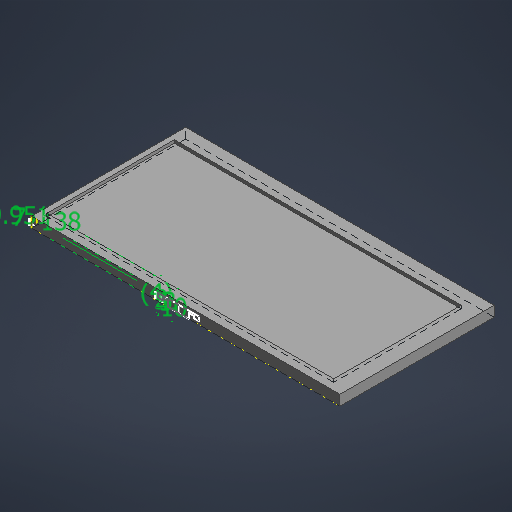
# Autodesk Inventor part: tray_multipart
Saved by Autodesk Inventor 2026 (Build 300175050, 175E)
## iProperties
Part Number: tray_multipart
Material: Generic
Document SubType Name: Modeling
Designer: romanov
Appearance: Default
Author: romanov
Autodesk Inventor part; units mm, degrees
ref_plane "YZ Plane" through (0, 0, 0) normal (1, 0, 0) x (0, 1, 0)
ref_plane "XZ Plane" through (0, 0, 0) normal (0, 1, 0) x (-1, 0, 0)
ref_plane "XY Plane" through (0, 0, 0) normal (0, 0, 1) x (1, 0, 0)
sketch "Sketch1" plane through (0, 0, 0) normal (0, 1, 0) x (-1, 0, 0)
  line L0 (150, 75) -> (-150, 75)
  line L1 (-150, 75) -> (-150, -75)
  line L2 (-150, -75) -> (150, -75)
  line L3 (150, -75) -> (150, 75)
  line L4 (150, 75) -> (-150, -75) construction
  line L5 (-150, 75) -> (150, -75) construction
  point P0 (0, 0)
  dimension "d0" = 300
  dimension "d1" = 150
  constraints: 12 end point, 2 midpoint, 2 parallel, 1 horizontal, 1 perpendicular
  measures "d0" distance between parallel lines of L1 L3
  measures "d1" distance between parallel lines of L0 L2
extrude "Extrusion1" add sketch "Sketch1" along normal blind 10
sketch "Sketch3" plane through (0, 10, 0) normal (0, 1, 0) x (1, 0, 0)
  line L0 (-145, -65) -> (134, -65)
  line L1 (134, -65) -> (134, 59)
  line L2 (134, 59) -> (-145, 59)
  line L3 (-145, 59) -> (-145, -65)
  line L4 (-150, 75) -> (-150, -75) projected
  line L5 (-150, -75) -> (150, -75) projected
  point P0 (0, 0)
  dimension "d4" = 279
  dimension "d5" = 124
  dimension "d6" = 5
  dimension "d7" = 10
  constraints: 8 end point, 2 parallel, 1 horizontal, 1 perpendicular
  measures "d4" distance of L1.end L2.end
  measures "d5" distance of L0.end L1.end
  measures "d6" distance between parallel lines of L4 L3
  measures "d7" distance between parallel lines of L5 L0
extrude "Extrusion2" cut sketch "Sketch3" against normal blind 3
sketch "Sketch5" plane through (-150, 0, 75) normal (0, 0, 1) x (1, 0, 0)
  line L0 (300, 0) -> (0, 0) construction
  line L1 (143, 0) -> (143, 9.9509) construction
  line L2 (0, 0) -> (0, 10) projected
  line L3 (123, 7) -> (123, 3)
  line L4 (123, 3) -> (128, 3)
  line L5 (128, 3) -> (128, 5)
  line L6 (128, 5) -> (133, 5)
  line L7 (133, 5) -> (133, 0)
  line L8 (133, 0) -> (143, 0)
  line L9 (123, 7) -> (143, 7)
  line L10 (163, 7) -> (163, 3)
  line L11 (163, 3) -> (158, 3)
  line L12 (158, 3) -> (158, 5)
  line L13 (158, 5) -> (153, 5)
  line L14 (153, 5) -> (153, 0)
  line L15 (153, 0) -> (143, 0)
  line L16 (163, 7) -> (143, 7)
  line L17 (143, 7) -> (143, 0)
  line L18 (5, 10) -> (5, 7) projected
  point P0 (0, 5)
  point P1 (128, 4)
  point P2 (123, 5)
  dimension "d20" = 2
  dimension "d23" = 5
  dimension "d24" = 5
  dimension "d25" = 2
  dimension "d26" = 4
  dimension "d27" = 10
  dimension "d28" = 138
  dimension "d29" = 7
  dimension "d30" = 9.9509
  constraints: 32 end point, 6 symmetric about line, 4 perpendicular, 3 midpoint, 3 point on line, 2 collinear, 1 horizontal, 1 vertical
  measures "d20" distance between parallel lines of L6 L4
  measures "d23" distance between parallel lines of L7 L5
  measures "d24" distance of L3.end L4.end
  measures "d25" distance between parallel lines of L9 L6
  measures "d26" distance of L3.start L3.end
  measures "d27" distance between parallel lines of L1 L7
  measures "d28" distance between parallel lines of L18 L1
  measures "d29" distance between parallel lines of L0 L9
  measures "d30" distance from line of L1.end L0
equation "\"d4\" = pebble_width"
equation "\"d5\" = pebble_height"
equation "\"pebble_height\" = 124"
equation "\"pebble_width\" = 279"
equation "\"pebble_depth\" = 16"
body "Solid1"
